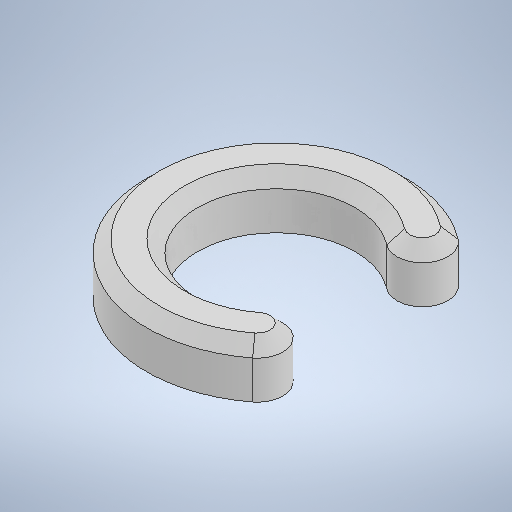
# Autodesk Inventor part: C_clip
Saved by Autodesk Inventor 2025.2 (Build 292293000, 293)
## iProperties
Created: 2025-02-02
Part Number: C_clip
Material: Generic
Document SubType Name: Modeling
Designer: mnguyen6
Density: 1 g/cm^3
Appearance: Default
Author: mnguyen6
Autodesk Inventor part; units mm, degrees
ref_plane "YZ Plane" through (0, 0, 0) normal (1, 0, 0) x (0, 1, 0)
ref_plane "XZ Plane" through (0, 0, 0) normal (0, 1, 0) x (-1, 0, 0)
ref_plane "XY Plane" through (0, 0, 0) normal (0, 0, 1) x (1, 0, 0)
sketch "Sketch1" plane through (0, 0, 0) normal (0, 1, 0) x (-1, 0, 0)
  circle A0 centre (0, 0) radius 3.1
  circle A1 centre (0, 0) radius 5.1
  circle A2 centre (-2.5, -3.2496) radius 1
  line L0 (0, 0) -> (-2.3308, 0) construction
  circle A3 centre (-2.5, 3.2496) radius 1
  point P0 (-1.8902, 2.457)
  point P1 (-1.8902, -2.457)
  point P2 (-3.1098, -4.0422)
  point P3 (-3.1098, 4.0422)
  dimension "d0" = 6.2
  dimension "d1" = 2
  dimension "d3" = 2.5
  constraints: 4 centre point, 2 end point, 2 tangent, 1 coincident, 1 horizontal, 1 symmetric about line, 1 other
  measures "d0" diameter of A0
  measures "d1" radial gap between concentric circles of A0 A1
  measures "d3" horizontal distance of L0.start A2.centre
extrude "Extrusion1" add sketch "Sketch1" along normal blind 2 contours A0 A3 A1 A2 | A3 | A2 picked at (4.3816, -0.4163)
chamfer "Chamfer1" distance 0.5 angle 45 4 edges at (-3.1, 2, 0) (3.2926, 2, -2.6399) (-5.1, 2, 0) (3.2926, 2, 2.6399)
body "Solid1"
